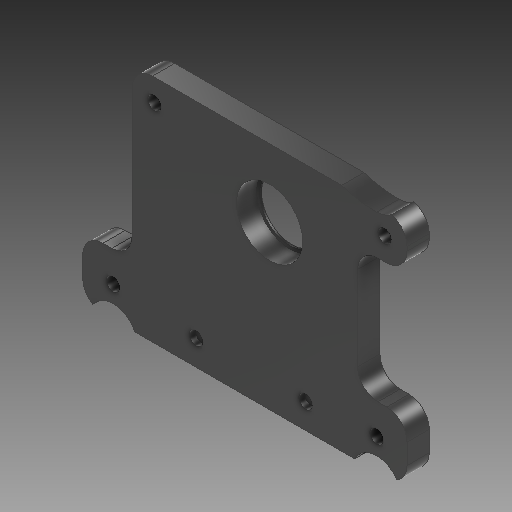
# Autodesk Inventor part: Extruder Mount Plate 2
Saved by Autodesk Inventor 2020.2 (Build 242310000, 310)
## iProperties
Created: 2020-03-20
Part Number: Extruder Mount Plate 2
Material: ABS Plastic
Document SubType Name: Modeling
Designer: rah75
Density: 1.06 g/cm^3
Appearance: Satin - Black
Author: rah75
Title: Extruder Back Plate
Autodesk Inventor part; units mm, degrees
ref_plane "YZ Plane" through (0, 0, 0) normal (1, 0, 0) x (0, 1, 0)
ref_plane "XZ Plane" through (0, 0, 0) normal (0, 1, 0) x (-1, 0, 0)
ref_plane "XY Plane" through (0, 0, 0) normal (0, 0, 1) x (1, 0, 0)
sketch "Sketch1" plane through (0, 0, 0) normal (0, 0, 1) x (1, 0, 0)
  line L0 (-40, -28.4) -> (40, -28.4)
  line L1 (40, -28.4) -> (40, 28.4)
  line L2 (40, 28.4) -> (-40, 28.4)
  line L3 (-40, 28.4) -> (-40, -28.4)
  line L4 (-40, -28.4) -> (40, 28.4) construction
  line L5 (40, -28.4) -> (-40, 28.4) construction
  line L6 (-32.5, -20.9) -> (32.5, -20.9) construction
  line L7 (32.5, -20.9) -> (32.5, 20.9) construction
  line L8 (32.5, 20.9) -> (-32.5, 20.9) construction
  line L9 (-32.5, 20.9) -> (-32.5, -20.9) construction
  line L10 (-32.5, -20.9) -> (32.5, 20.9) construction
  line L11 (32.5, -20.9) -> (-32.5, 20.9) construction
  circle A0 centre (-32.5, -20.9) radius 3.25 construction
  circle A1 centre (32.5, 20.9) radius 3.25 construction
  circle A2 centre (32.5, -20.9) radius 3.25 construction
  line L12 (-40, -13.4) -> (-27.8, -13.4)
  line L13 (-27.8, -13.4) -> (-27.8, 28.4)
  circle A3 centre (-20.3, 20.9) radius 3.25 construction
  line L14 (40, 28.4) -> (32.5, 20.9)
  line L15 (-27.8, 28.4) -> (-20.3, 20.9) construction
  point P0 (0, 0)
  point P1 (34.5, 22.9)
  point P2 (-22.3, 22.9)
  dimension "d0" = 80
  dimension "d1" = 56.8
  dimension "d2" = 41.8
  dimension "d3" = 65
  dimension "d4" = 6.5
  dimension "d5" = 6.5
  dimension "d6" = 6.5
  dimension "d8" = 7.5
  dimension "d9" = 7.5
  dimension "d10" = 7.5
  dimension "d11" = 12.2
  dimension "d12" = 6.5
  dimension "d13" = 7.5
  dimension "d61" = 5.5
  dimension "d62" = 5.5
  constraints: 32 end point, 5 point on line, 4 centre point, 4 midpoint, 4 parallel, 3 coincident, 3 horizontal, 3 perpendicular
  measures "d0" distance of L2.end L1.end
  measures "d1" distance of L1.end L0.end
  measures "d2" distance of L7.end L6.end
  measures "d3" distance of L7.end L8.end
  measures "d4" diameter of A0
  measures "d5" diameter of A1
  measures "d6" diameter of A2
  measures "d8" distance between parallel lines of L3 L9
  measures "d9" distance between parallel lines of L8 L2
  measures "d10" distance from line of L6.start L12
  measures "d11" distance between parallel lines of L3 L13
  measures "d12" diameter of A3
  measures "d13" distance from line of L13 L15.end
  measures "d61" distance from line of point (34.5, 22.9) L1
  measures "d62" distance from line of L13 point (-22.3, 22.9)
extrude "Base" add sketch "Sketch1" against normal blind 5.5 contours L3 L12 L13 L2 L1 L0
hole "Mounting Holes" at (32.5, -20.9, 0) at (-32.5, -20.9, 0) at (34.5, 22.9, 0) at (-22.3, 22.9, 0) direction (0, 0, -1) diameter 3.4 end through all clearance for "Socket Head Cap Screw" size "M3" standard "Ansi Metric M Profile"
fillet "Fillet1" radius 5 6 edges at (-40, -28.4, -2.75) (-40, -13.4, -2.75) (-27.8, -13.4, -2.75) (-27.8, 28.4, -2.75) (40, 28.4, -2.75) (40, -28.4, -2.75)
sketch "Sketch2" plane through (0, 0, 0) normal (0, 0, 1) x (1, 0, 0)
  circle A0 centre (32.5, -20.9) radius 1.7 projected
  point P0 (0, 0)
  point P1 (6.1, -6.4)
  point P2 (6.1, 11.6)
  dimension "d24" = 6.1
  dimension "d26" = 18
  dimension "d63" = 14.5
  constraints: 1 vertical alignment
  measures "d24" horizontal distance of point (6.1, -6.4) point (0, 0)
  measures "d26" distance of point (6.1, -6.4) point (6.1, 11.6)
  measures "d63" vertical distance of A0.centre point (6.1, -6.4)
hole "Bearing Bore" at (6.1, 11.6, 0) direction (0, 0, -1) diameter 15 end through all counterbore diameter 16.4 counterbore depth 5
sketch "Sketch8" plane through (0, 0, 0) normal (0, 0, 1) x (1, 0, 0)
  line L0 (27.8, 17.4) -> (40, 17.4)
  line L1 (40, 17.4) -> (40, -13.4)
  line L2 (40, -13.4) -> (27.8, -13.4)
  line L3 (27.8, -13.4) -> (27.8, 17.4)
  line L4 (27.8, 17.4) -> (40, -13.4) construction
  line L5 (40, 17.4) -> (27.8, -13.4) construction
  circle A0 centre (34.5, 22.9) radius 1.7 projected
  circle A1 centre (32.5, -20.9) radius 1.7 projected
  line L6 (40, -23.4) -> (40, 23.4) projected
  line L7 (-35, -28.4) -> (35, -28.4) projected
  point P0 (0, 0)
  point P1 (33.9, 2)
  dimension "d73" = 12.2
  dimension "d77" = 15
  dimension "d78" = 7.5
  dimension "d79" = 5.5
  constraints: 12 end point, 2 midpoint, 2 parallel, 1 collinear, 1 horizontal, 1 perpendicular
  measures "d73" distance of L0.start L0.end
  measures "d77" distance between parallel lines of L7 L2
  measures "d78" distance from line of L2 A1.centre
  measures "d79" distance from line of L0 A0.centre
extrude "Clamp Clearance" cut sketch "Sketch8" against normal blind 10 contours L0 L1 L2 L3
fillet "Fillet3" radius 5 2 edges at (40, 17.4, -2.75) (40, -13.4, -2.75)
sketch "Sketch9" plane through (0, 0, -5.5) normal (0, 0, -1) x (-1, 0, 0)
  circle A0 centre (-34.5, 22.9) radius 1.7 projected
  arc A1 (-32.5, 33) -> (-22.5, 35.5) centre (-32.5, 54.25) ccw construction
  arc A2 (-32.5, 27) -> (-19.6765, 30.2059) centre (-32.5, 54.25) ccw
  arc A3 (-32.5, 39) -> (-25.3235, 40.7941) centre (-32.5, 54.25) ccw
  arc A4 (-32.5, 39) -> (-32.5, 27) centre (-32.5, 33) ccw
  arc A5 (-19.6765, 30.2059) -> (-25.3235, 40.7941) centre (-22.5, 35.5) ccw
  circle A6 centre (-32.5, -31) radius 6
  circle A7 centre (32.5, -31) radius 6
  circle A8 centre (-32.5, -20.9) radius 1.7 projected
  circle A9 centre (32.5, -20.9) radius 1.7 projected
  point P0 (0, 0)
  dimension "d80" = 2
  dimension "d81" = 10.1
  dimension "d82" = 6
  dimension "d83" = 10
  dimension "d84" = 2.5
  dimension "d85" = 15.25
  dimension "d86" = 10.1
  dimension "d87" = 10.1
  dimension "d88" = 12
  constraints: 10 point on circle, 7 centre point, 4 tangent, 2 vertical alignment, 1 equal radius
  measures "d80" horizontal distance of A0.centre A1.start
  measures "d81" vertical distance of A0.centre A1.start
  measures "d82" radius of A4
  measures "d83" horizontal distance of A1.end A1.start
  measures "d84" vertical distance of A1.start A1.end
  measures "d85" radius of A3
  measures "d86" distance of A9.centre A7.centre
  measures "d87" distance of A6.centre A8.centre
  measures "d88" diameter of A6
extrude "Bolt Clearance" cut sketch "Sketch9" against normal blind 10 contours A4 A3 A5 A2 | A6 | A7
sketch "Sketch10" plane through (0, 0, -5.5) normal (0, 0, -1) x (-1, 0, 0)
  line L0 (-27.0926, -28.4) -> (27.0926, -28.4) projected
  circle A0 centre (-6.1, 11.6) radius 7.5 projected
  point P0 (0, 0)
  point P1 (-15, -22.2)
  point P2 (12, -22.2)
  dimension "d91" = 6.2
  dimension "d92" = 6.2
  dimension "d102" = 15
  dimension "d103" = 12
  measures "d91" distance from line of L0 point (-15, -22.2)
  measures "d92" distance from line of L0 point (12, -22.2)
  measures "d102" horizontal distance of point (-15, -22.2) point (0, 0)
  measures "d103" horizontal distance of point (12, -22.2) point (0, 0)
hole "Lower Block Holes" at (15, -22.2, -5.5) at (-12, -22.2, -5.5) direction (0, 0, 1) diameter 3.4 end through all counterbore diameter 6.5 counterbore depth 3 clearance for "Socket Head Cap Screw" size "M3" standard "Ansi Metric M Profile"
sketch "Sketch11" plane through (15, -22.2, -2.5) normal (0, 0, -1) x (-1, 0, 0)
  circle A0 centre (0, 0) radius 1.7 projected
  circle A1 centre (27, 0) radius 1.7 projected
  point P0 (15, 22.2)
extrude "Print Feature" add sketch "Sketch11" against normal blind 1
fillet "Fillet4" radius 5 2 edges at (27.8, -13.4, -2.75) (27.8, 17.4, -2.75)
equation "\"d13\" = d10"
body "Solid1"
